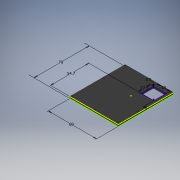
# Autodesk Inventor part: Lid
Saved by Autodesk Inventor 2019.4 (Build 234330000, 330)
## iProperties
Created: 2020-06-11
Part Number: Lid
Material: Generic
Document SubType Name: Modeling
Designer: ions
Density: 1 g/cm^3
Appearance: Default
Author: ions
Autodesk Inventor part; units mm, degrees
ref_plane "YZ Plane" through (0, 0, 0) normal (1, 0, 0) x (0, 1, 0)
ref_plane "XZ Plane" through (0, 0, 0) normal (0, 1, 0) x (-1, 0, 0)
ref_plane "XY Plane" through (0, 0, 0) normal (0, 0, 1) x (1, 0, 0)
sketch "Sketch1" plane through (0, 0, 0) normal (0, 1, 0) x (-1, 0, 0)
  line L0 (43.0361, 44.0554) -> (-25.9639, 44.0554)
  line L1 (-25.9639, 44.0554) -> (-25.9639, -34.9446)
  line L2 (-25.9639, -34.9446) -> (43.0361, -34.9446)
  line L3 (43.0361, -34.9446) -> (43.0361, 44.0554)
  point P0 (0, 0)
  dimension "d0" = 69
  dimension "d1" = 79
  constraints: 8 end point, 2 parallel, 1 horizontal, 1 perpendicular
  measures "d0" distance between parallel lines of L1 L3
  measures "d1" distance between parallel lines of L2 L0
extrude "Extrusion1" add sketch "Sketch1" along normal blind 2.5
sketch "Sketch2" plane through (0, 2.5, 0) normal (0, 1, 0) x (1, 0, 0)
  circle A0 centre (23.9639, -42.0554) radius 1.2843
  line L0 (25.9639, -44.0554) -> (25.9639, 34.9446) projected
  line L1 (-43.0361, -44.0554) -> (25.9639, -44.0554) projected
  circle A1 centre (-41.0361, 2.9446) radius 1.3818
  circle A2 centre (23.9639, -14.0554) radius 1.5724
  line L2 (-43.0361, 34.9446) -> (-43.0361, -44.0554) projected
  line L3 (25.9639, 34.9446) -> (-43.0361, 34.9446) projected
  circle A3 centre (-8.5361, 32.9446) radius 1.5869
  circle A4 centre (-8.5361, -42.0554) radius 2.0414
  point P0 (0, 0)
  dimension "d4" = 2
  dimension "d5" = 2
  dimension "d26" = 2
  dimension "d27" = 2
  dimension "d28" = 32
  dimension "d29" = 30
  dimension "d37" = 2
  dimension "d38" = 2
  dimension "d39" = 34.5
  dimension "d40" = 34.5
  constraints: 5 centre point
  measures "d4" distance from line of A0.centre L0
  measures "d5" distance from line of A0.centre L1
  measures "d26" distance from line of A1.centre L2
  measures "d27" distance from line of L0 A2.centre
  measures "d28" distance from line of L3 A1.centre
  measures "d29" distance from line of L1 A2.centre
  measures "d37" distance from line of L3 A3.centre
  measures "d38" distance from line of L1 A4.centre
  measures "d39" distance from line of A3.centre L2
  measures "d40" distance from line of A4.centre L2
hole "Hole1" at (23.9639, 2.5, 42.0554) direction (0, -1, 0) diameter 2.3 end through all counterbore diameter 3.3 counterbore depth 1.25
pattern_linear "Rectangular Pattern1" count 2 spacing 65 along (-1, 0, 0) count 2 spacing 75 along (0, 0, -1) of "Hole1"
sketch "Sketch3" plane through (0, 2.5, 0) normal (0, 1, 0) x (1, 0, 0)
  line L0 (5.4639, 28.1446) -> (20.4639, 28.1446)
  line L1 (21.9639, 26.6446) -> (21.9639, 12.1446)
  line L2 (20.4639, 10.6446) -> (5.4639, 10.6446)
  line L3 (3.9639, 12.1446) -> (3.9639, 26.6446)
  line L4 (-43.0361, -44.0554) -> (25.9639, -44.0554) projected
  line L5 (25.9639, -44.0554) -> (25.9639, 34.9446) projected
  arc A0 (5.4639, 28.1446) -> (3.9639, 26.6446) centre (5.4639, 26.6446) ccw
  arc A1 (21.9639, 26.6446) -> (20.4639, 28.1446) centre (20.4639, 26.6446) ccw
  arc A2 (20.4639, 10.6446) -> (21.9639, 12.1446) centre (20.4639, 12.1446) ccw
  arc A3 (3.9639, 12.1446) -> (5.4639, 10.6446) centre (5.4639, 12.1446) ccw
  point P0 (0, 0)
  point P1 (3.9639, 28.1446)
  point P2 (21.9639, 10.6446)
  point P3 (21.9639, 28.1446)
  point P4 (3.9639, 10.6446)
  dimension "d19" = 54.7
  dimension "d20" = 4
  dimension "d21" = 18
  dimension "d22" = 17.5
  dimension "d25" = 1.5
  constraints: 8 end point, 8 point on circle, 8 point on line, 8 tangent, 4 centre point, 3 equal radius, 2 parallel, 1 horizontal, 1 perpendicular
  measures "d19" distance between parallel lines of L2 L4
  measures "d20" distance between parallel lines of L5 L1
  measures "d21" distance between parallel lines of L3 L1
  measures "d22" distance between parallel lines of L2 L0
  measures "d25" radius of A0
extrude "Extrusion2" cut sketch "Sketch3" against normal blind 2.5
hole "Hole2" at (-41.0361, 2.5, -2.9446) at (23.9639, 2.5, 14.0554) direction (0, -1, 0) diameter 2.3 end through all counterbore diameter 3.3 counterbore depth 1.25
hole "Hole3" at (-8.5361, 2.5, -32.9446) at (-8.5361, 2.5, 42.0554) direction (0, -1, 0) diameter 2.3 end through all counterbore diameter 3.3 counterbore depth 1.25
body "Solid1"
